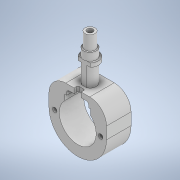
# Autodesk Inventor part: Fahrwerk_motorhalterung
Saved by Autodesk Inventor 2021 (Build 250183000, 183)
## iProperties
Created: 2020-12-29
Part Number: Fahrwerk_motorhalterung
Material: Generisch
Document SubType Name: Modeling
Designer: laure
Density: 1 g/cm^3
Appearance: Vorgabe
Author: laure
## iProperties of the stored document _3D-Druck.ipt
Created: 2020-12-29
Part Number: _3D-Druck
Material: Generisch
Document SubType Name: Modeling
Designer: laure
Density: 1 g/cm^3
Appearance: Vorgabe
Author: laure
Autodesk Inventor part; units mm, degrees
ref_plane "YZ Plane" through (0, 0, 0) normal (1, 0, 0) x (0, 1, 0)
ref_plane "XZ Plane" through (0, 0, 0) normal (0, 1, 0) x (-1, 0, 0)
ref_plane "XY Plane" through (0, 0, 0) normal (0, 0, 1) x (1, 0, 0)
sketch "Skizze1" plane through (0, 0, 0) normal (0, 0, 1) x (1, 0, 0)
  circle A0 centre (17.75, 0) radius 1.75
  circle A1 centre (-17.75, 0) radius 1.75
  circle A2 centre (0, 0) radius 14.25
  arc A3 (-22.25, 0) -> (22.25, 0) centre (0, 0) ccw
  line L0 (-22.25, 25.25) -> (22.25, 25.25)
  line L1 (22.25, 25.25) -> (22.25, 22.25)
  line L2 (22.25, 22.25) -> (-22.25, 22.25)
  line L3 (-22.25, 22.25) -> (-22.25, 25.25)
  line L4 (0, -31.75) -> (0, 34.75) projected
  line L5 (-22.25, 22.25) -> (-22.25, 0)
  line L6 (22.25, 22.25) -> (22.25, 0)
  dimension "d2" = 3.5
  dimension "d3" = 3.5
  dimension "d8" = 28.5
  dimension "d9" = 44.5
  dimension "d10" = 44.5
  dimension "d11" = 3
  constraints: 12 end point, 4 centre point, 2 parallel, 2 point on circle, 2 tangent, 1 coincident, 1 horizontal, 1 perpendicular, 1 other
  measures "d2" diameter of A0
  measures "d3" diameter of A1
  measures "d8" diameter of A2
  measures "d9" diameter of A3
  measures "d10" distance between parallel lines of L1 L3
  measures "d11" distance between parallel lines of L2 L0
extrude "Extrusion2" add sketch "Skizze1" along normal mid plane 19 contours A2 L4 L2 L6 A3 | A2 L4 A3 L5 L2
sketch "Skizze2" plane through (0, 0, 9.5) normal (0, 0, 1) x (1, 0, 0)
  line L0 (-8.5, 18.4) -> (8.5, 18.4)
  line L1 (8.5, 18.4) -> (8.5, 11.4)
  line L2 (8.5, 11.4) -> (-8.5, 11.4)
  line L3 (0, -31.15) -> (0, 31.15) projected
  line L4 (-31.15, 0) -> (31.15, 0) projected
  line L5 (-10, 14.5) -> (-8.5, 14.5)
  line L6 (-10, 14.5) -> (-10, 10)
  line L7 (-10, 10) -> (-8.5, 10)
  line L8 (-8.5, 18.4) -> (-8.5, 11.4)
  line L9 (-8.5, 14.5) -> (-8.5, 10)
  line L10 (10, 14.5) -> (8.5, 14.5)
  line L11 (10, 14.5) -> (10, 10)
  line L12 (10, 10) -> (8.5, 10)
  line L13 (8.5, 14.5) -> (8.5, 10)
  point P0 (0, 0)
  point P1 (0, 11.4)
  point P2 (0, 18.4)
  dimension "d14" = 17
  dimension "d15" = 7
  dimension "d16" = 11.4
  dimension "d34" = 1.5
  dimension "d45" = 4.5
  dimension "d46" = 10
  dimension "d48" = 1.5
  constraints: 24 end point, 4 symmetric about line, 2 perpendicular, 2 vertical, 1 collinear, 1 horizontal, 1 parallel, 1 other
  measures "d14" distance of L1.end L2.end
  measures "d15" distance of L0.end L1.end
  measures "d16" distance between parallel lines of L4 L2
  measures "d34" distance of L5.start L5.end
  measures "d45" distance between parallel lines of L5 L7
  measures "d46" distance between parallel lines of L4 L7
  measures "d48" distance between parallel lines of L8 L6
extrude "Extrusion3" cut sketch "Skizze2" against normal blind 19
sketch "Skizze3" plane through (-8.5, 18.4, 9.5) normal (0, -1, 0) x (1, 0, 0)
  line L0 (0, 0) -> (17, 0) projected
  line L1 (5.75, 0) -> (11.25, 0)
  line L2 (11.25, 0) -> (11.25, -3)
  line L3 (11.25, -3) -> (5.75, -3)
  line L4 (5.75, -3) -> (5.75, 0)
  line L5 (0, 0) -> (0, -19) projected
  point P0 (8.5, -9.5)
  dimension "d19" = 5.5
  dimension "d20" = 3
  dimension "d38" = 5.75
  constraints: 8 end point, 2 parallel, 1 horizontal, 1 perpendicular, 1 point on line
  measures "d19" distance of L2.end L3.end
  measures "d20" distance between parallel lines of L0 L3
  measures "d38" distance between parallel lines of L4 L5
extrude "Extrusion4" cut sketch "Skizze3" against normal blind 4
fillet "Rundung1" radius 2 2 edges at (-8.5, 18.4, 0) (8.5, 18.4, 0)
sketch "Skizze4" plane through (-22.25, 22.25, -9.5) normal (0, 1, 0) x (1, 0, 0)
  line L0 (0, -19) -> (0, 0) projected
  line L1 (0, 0) -> (44.5, 0) projected
  line L2 (44.5, -19) -> (0, -19) projected
  line L3 (44.5, 0) -> (44.5, -19) projected
  circle A0 centre (22.25, -9.5) radius 4.9
  point P0 (25, -19)
  dimension "d39" = 9.8
  constraints: 1 centre point, 1 coincident
  measures "d39" diameter of A0
fillet "Rundung2" radius 1 2 edges at (-2.75, 20.325, 6.5) (2.75, 20.325, 6.5)
extrude "Extrusion7" add sketch "Skizze4" along normal blind 15 contours A0
sketch "Skizze5" plane through (0, 37.25, 0) normal (0, 1, 0) x (1, 0, 0)
  circle A0 centre (0, 0) radius 6.5
  dimension "d51" = 13
  constraints: 1 centre point, 1 coincident
  measures "d51" diameter of A0
extrude "Extrusion8" add sketch "Skizze5" along normal blind 3
sketch "Skizze6" plane through (0, 40.25, 0) normal (0, 1, 0) x (1, 0, 0)
  circle A0 centre (0, 0) radius 5
  dimension "d54" = 10
  constraints: 1 centre point, 1 coincident
  measures "d54" diameter of A0
extrude "Extrusion9" add sketch "Skizze6" along normal blind 6
sketch "Skizze8" plane through (0, 40.25, 0) normal (0, 1, 0) x (1, 0, 0)
  line L0 (-6.5, 9.5) -> (-6.5, -9.5) projected
  line L1 (6.5, -9.5) -> (6.5, 9.5) projected
  line L2 (-6.5, 0) -> (6.5, 0)
  line L3 (6.5, 0) -> (6.5, -6.5)
  line L4 (6.5, -6.5) -> (-6.5, -6.5)
  line L5 (-6.5, -6.5) -> (-6.5, 0)
  line L6 (-6.5, -6.5) -> (6.5, -6.5)
  line L7 (6.5, -6.5) -> (6.5, -4.5)
  line L8 (6.5, -4.5) -> (-6.5, -4.5)
  line L9 (-6.5, -4.5) -> (-6.5, -6.5)
  point P0 (0, 0)
  point P1 (-6.5, -4.5)
  point P2 (-6.5, -6.5)
  dimension "d60" = 6.5
  dimension "d61" = 2
  constraints: 16 end point, 4 parallel, 2 horizontal, 2 perpendicular, 2 point on line, 1 midpoint
  measures "d60" distance of L2.end L3.end
  measures "d61" distance of L7.end L6.end
sketch "Skizze9" plane through (0, 46.25, 0) normal (0, 1, 0) x (1, 0, 0)
  circle A0 centre (0, 0) radius 3.9
  dimension "d62" = 7.8
  constraints: 1 centre point, 1 coincident
  measures "d62" diameter of A0
extrude "Extrusion11" add sketch "Skizze9" along normal blind 11
sketch "Skizze10" plane through (0, 57.25, 0) normal (0, 1, 0) x (1, 0, 0)
  circle A0 centre (0, 0) radius 2.25
  dimension "d65" = 4.5
  constraints: 1 centre point, 1 coincident
  measures "d65" diameter of A0
extrude "Extrusion12" cut sketch "Skizze10" against normal blind 6
extrude "Extrusion13" cut sketch "Skizze8" against normal blind 18 contours L8 L1 L4 L0
fillet "Rundung6" radius 13 2 edges at (-22.25, 22.25, 0) (22.25, 22.25, 0)
